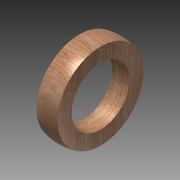
# Autodesk Inventor part: bigWheel_01
Saved by Autodesk Inventor 2013 (Build 170138000, 138)
## iProperties
Created: 2013-01-08
Part Number: bigWheel_01
Material: Wood (Maple)
Document SubType Name: Modeling
Designer: Nano
Density: 0.57 g/cm^3
Mass: 2208.67 g
Surface Area: 1950.19 cm^2
Volume: 3874.85 cm^3
Author: Nano
Autodesk Inventor part; units mm, degrees
ref_plane "YZ Plane" through (0, 0, 0) normal (1, 0, 0) x (0, 1, 0)
ref_plane "XZ Plane" through (0, 0, 0) normal (0, 1, 0) x (-1, 0, 0)
ref_plane "XY Plane" through (0, 0, 0) normal (0, 0, 1) x (1, 0, 0)
sketch "Sketch1" plane through (0, 0, 0) normal (0, 0, 1) x (1, 0, 0)
  circle A0 centre (0, 0) radius 146.05
  line L0 (0, 146.05) -> (234.2216, 146.05) construction
  line L1 (-34.925, 196.85) -> (34.925, 196.85) construction
  line L2 (34.925, 196.85) -> (34.925, 95.25)
  line L3 (34.925, 95.25) -> (-34.925, 95.25)
  line L4 (-34.925, 95.25) -> (-34.925, 196.85)
  line L5 (-34.925, 196.85) -> (34.925, 95.25) construction
  line L6 (34.925, 196.85) -> (-34.925, 95.25) construction
  line L7 (0, 0) -> (253.8576, 0) construction
  point P0 (-34.925, 141.8127)
  point P1 (34.925, 141.8127)
  dimension "d6" = 292.1
  dimension "d7" = 69.85
  dimension "d8" = 101.6
  dimension "d9" = 95.25
  constraints: 16 end point, 3 point on circle, 2 horizontal, 2 midpoint, 2 parallel, 2 perpendicular, 2 point on line, 1 centre point, 1 tangent, 1 other
  measures "d6" diameter of A0
  measures "d7" distance of L2.end L3.end
  measures "d8" distance of L1.end L2.end
  measures "d9" distance from line of L7.start L3
revolve "Revolution2" add sketch "Sketch1" angle 360 about axis through (0, 0, 0) along (1, 0, 0) picked at (2.3502, 112.1266) contours L2 L3 L4 A0
sketch "Sketch4" plane through (-34.925, 0, 0) normal (-1, 0, 0) x (0, 0, 1)
  circle A0 centre (0, 0) radius 95.25 projected
  circle A1 centre (0, 0) radius 117.475
  dimension "d24" = 234.95
  constraints: 1 centre point, 1 coincident
  measures "d24" diameter of A1
extrude "Extrusion3" cut sketch "Sketch4" against normal blind 12.7
body "Solid2"
